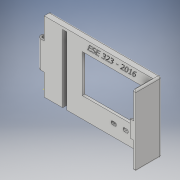
# Autodesk Inventor part: case top_new
Saved by Autodesk Inventor 2017 (Build 210142000, 142)
## iProperties
Created: 2016-12-08
Part Number: case top_new
Material: Generic
Document SubType Name: Modeling
Designer: radrajith
Density: 1 g/cm^3
Appearance: Default
Author: radrajith
Autodesk Inventor part; units mm, degrees
ref_plane "YZ Plane" through (0, 0, 0) normal (1, 0, 0) x (0, 1, 0)
ref_plane "XZ Plane" through (0, 0, 0) normal (0, 1, 0) x (-1, 0, 0)
ref_plane "XY Plane" through (0, 0, 0) normal (0, 0, 1) x (1, 0, 0)
sketch "Sketch1" plane through (0, 0, 0) normal (0, 0, 1) x (1, 0, 0)
  line L0 (0, 0) -> (138.5, 0)
  line L1 (138.5, 0) -> (138.5, 83)
  line L2 (138.5, 83) -> (0, 83)
  line L3 (0, 83) -> (0, 0)
  dimension "d0" = 138.5
  dimension "d1" = 83
  constraints: 8 end point, 2 parallel, 1 horizontal, 1 perpendicular
  measures "d0" distance of L2.end L1.end
  measures "d1" distance of L1.end L0.end
extrude "Extrusion1" add sketch "Sketch1" along normal blind 8
sketch "Sketch2" plane through (0, 0, 8) normal (0, 0, 1) x (1, 0, 0)
  line L0 (138.5, 0) -> (138.5, 83) projected
  line L1 (0, 0) -> (138.5, 0) projected
  line L2 (138.5, 83) -> (136, 83)
  line L3 (136, 83) -> (136, 0)
  line L4 (136, 0) -> (138.5, 0)
  line L5 (138.5, 0) -> (138.5, 83)
  line L6 (0, 83) -> (0, 0) projected
  dimension "d15" = 136
  constraints: 8 end point, 2 parallel, 1 horizontal, 1 perpendicular, 1 point on line
  measures "d15" distance between parallel lines of L3 L6
extrude "Extrusion2" add sketch "Sketch2" along normal blind 22.5
sketch "Sketch3" plane through (136, 0, 8) normal (-1, 0, 0) x (0, 0, 1)
  line L0 (22.5, 0) -> (22.5, 83) projected
  line L1 (22.5, 31.3) -> (20.7, 31.3)
  line L2 (20.7, 31.3) -> (20.7, 51)
  line L3 (20.7, 51) -> (22.5, 51)
  line L4 (22.5, 51) -> (22.5, 31.3)
  point P0 (-8, 0)
  dimension "d6" = 1.8
  constraints: 8 end point, 2 parallel, 1 horizontal, 1 perpendicular, 1 point on line
  measures "d6" distance of L2.end L3.end
extrude "Extrusion3" add sketch "Sketch3" along normal blind 4
sketch "Sketch5" plane through (0, 0, 8) normal (0, 0, 1) x (1, 0, 0)
  line L0 (0, 0) -> (138.5, 0) projected
  line L1 (0, 0) -> (8, 0)
  line L2 (8, 0) -> (8, 25.5)
  line L3 (8, 25.5) -> (0, 25.5)
  line L4 (0, 25.5) -> (0, 0)
  line L5 (0, 83) -> (0, 0) projected
  line L6 (0, 83) -> (8, 83)
  line L7 (8, 83) -> (8, 57.5)
  line L8 (8, 57.5) -> (0, 57.5)
  line L9 (0, 57.5) -> (0, 83)
  dimension "d9" = 8
  dimension "d10" = 25.5
  dimension "d11" = 8
  dimension "d12" = 25.5
  constraints: 16 end point, 4 parallel, 2 horizontal, 2 perpendicular
  measures "d9" distance of L3.end L2.end
  measures "d10" distance of L2.end L1.end
  measures "d11" distance of L7.end L8.end
  measures "d12" distance of L6.end L7.end
extrude "Extrusion4" cut sketch "Sketch5" against normal blind 8
sketch "Sketch6" plane through (0, 25.5, 8) normal (0, -1, 0) x (1, 0, 0)
  circle A0 centre (4, -4) radius 2
  point P0 (0, -8)
  constraints: 1 centre point
extrude "Extrusion5" cut sketch "Sketch6" against normal blind 40
fillet "Fillet1" radius 4 2 edges at (0, 41.5, 8) (0, 41.5, 0)
sketch "Sketch7" plane through (0, 0, 0) normal (0, 0, -1) x (-1, 0, 0)
  line L0 (-115, 24) -> (-53, 24)
  line L1 (-53, 24) -> (-53, 69)
  line L2 (-53, 69) -> (-115, 69)
  line L3 (-115, 69) -> (-115, 24)
  line L4 (-8, 57.5) -> (-8, 83) projected
  line L5 (-138.5, 83) -> (-8, 83) projected
  point P0 (0, 0)
  dimension "d19" = 62
  dimension "d20" = 45
  dimension "d21" = 45
  dimension "d22" = 14
  constraints: 8 end point, 2 parallel, 1 horizontal, 1 perpendicular
  measures "d19" distance of L2.end L1.end
  measures "d20" distance of L1.end L0.end
  measures "d21" distance between parallel lines of L4 L1
  measures "d22" distance between parallel lines of L2 L5
extrude "Extrusion6" cut sketch "Sketch7" against normal blind 10
chamfer "Chamfer1" distance 5 angle 45 4 edges at (115, 46.5, 0) (84, 69, 0) (53, 46.5, 0) (84, 24, 0)
sketch "Sketch8" plane through (0, 0, 8) normal (0, 0, 1) x (1, 0, 0)
  line L0 (115, 69) -> (115, 24) projected
  line L1 (115, 69) -> (125, 69)
  line L2 (125, 69) -> (125, 24)
  line L3 (125, 24) -> (115, 24)
  line L4 (115, 24) -> (115, 69)
  point P0 (0, 0)
  dimension "d28" = 10
  constraints: 8 end point, 2 parallel, 1 horizontal, 1 perpendicular
  measures "d28" distance of L2.end L3.end
extrude "Extrusion7" cut sketch "Sketch8" against normal blind 5
sketch "Sketch9" plane through (0, 0, 8) normal (0, 0, 1) x (1, 0, 0)
  line L0 (8, 0) -> (138.5, 0) projected
  line L1 (34.5, 0) -> (29.7, 0)
  line L2 (29.7, 0) -> (29.7, 80)
  line L3 (29.7, 80) -> (34.5, 80)
  line L4 (34.5, 80) -> (34.5, 0)
  point P0 (0, 0)
  dimension "d31" = 4.8
  constraints: 8 end point, 2 parallel, 1 horizontal, 1 perpendicular, 1 point on line
  measures "d31" distance of L2.end L3.end
extrude "Extrusion8" cut sketch "Sketch9" against normal blind 5
sketch "Sketch10" plane through (0, 0, 8) normal (0, 0, 1) x (1, 0, 0)
  line L0 (29.7, 0) -> (29.7, 80) projected
  line L1 (34.5, 0) -> (29.7, 0)
  line L2 (29.7, 0) -> (29.7, 10)
  line L3 (29.7, 10) -> (34.5, 10)
  line L4 (34.5, 10) -> (34.5, 0)
  point P0 (0, 0)
  constraints: 8 end point, 2 parallel, 1 horizontal, 1 perpendicular, 1 point on line
extrude "Extrusion9" cut sketch "Sketch10" against normal blind 7.2
sketch "Sketch11" plane through (0, 0, 0) normal (0, 0, -1) x (-1, 0, 0)
  line L0 (-8, 0) -> (-138.5, 0) projected
  line L1 (-136, 0) -> (-136, 83) projected
  line L2 (-105.5, 16) -> (-102.5, 16)
  line L3 (-101, 14.5) -> (-101, 13.5)
  line L4 (-102.5, 12) -> (-105.5, 12)
  line L5 (-107, 13.5) -> (-107, 14.5)
  line L6 (-107, 16) -> (-101, 12) construction
  line L7 (-101, 16) -> (-107, 12) construction
  line L8 (-91.5, 16) -> (-88.5, 16)
  line L9 (-87, 14.5) -> (-87, 13.5)
  line L10 (-88.5, 12) -> (-91.5, 12)
  line L11 (-93, 13.5) -> (-93, 14.5)
  line L12 (-93, 16) -> (-87, 12) construction
  line L13 (-87, 16) -> (-93, 12) construction
  arc A0 (-91.5, 16) -> (-93, 14.5) centre (-91.5, 14.5) ccw
  arc A1 (-93, 13.5) -> (-91.5, 12) centre (-91.5, 13.5) ccw
  arc A2 (-88.5, 12) -> (-87, 13.5) centre (-88.5, 13.5) ccw
  arc A3 (-87, 14.5) -> (-88.5, 16) centre (-88.5, 14.5) ccw
  arc A4 (-101, 14.5) -> (-102.5, 16) centre (-102.5, 14.5) ccw
  arc A5 (-105.5, 16) -> (-107, 14.5) centre (-105.5, 14.5) ccw
  arc A6 (-107, 13.5) -> (-105.5, 12) centre (-105.5, 13.5) ccw
  arc A7 (-102.5, 12) -> (-101, 13.5) centre (-102.5, 13.5) ccw
  point P0 (0, 0)
  point P1 (-104, 14)
  point P2 (-90, 14)
  dimension "d47" = 6
  dimension "d48" = 4
  dimension "d49" = 6
  dimension "d50" = 4
  dimension "d51" = 1.5
  dimension "d52" = 32
  dimension "d53" = 46
  constraints: 24 end point, 16 point on circle, 16 point on line, 16 tangent, 8 centre point, 7 equal radius, 4 midpoint, 4 parallel, 2 horizontal, 2 perpendicular
  measures "d47" distance of L6.end L7.end
  measures "d48" distance of L7.start L6.end
  measures "d49" distance of L12.end L13.end
  measures "d50" distance of L13.start L12.end
  measures "d51" radius of A0
  measures "d52" distance from line of point (-104, 14) L1
  measures "d53" distance from line of point (-90, 14) L1
extrude "Extrusion10" cut sketch "Sketch11" against normal blind 8
fillet "Fillet3" radius 2 5 edges at (138.5, 41.5, 0) (8, 70.25, 0) (73.25, 83, 0) (73.25, 0, 0) (8, 12.75, 0)
fillet "Fillet4" radius 2 6 edges at (137.25, 83, 30.5) (137.25, 0, 30.5) (137.9142, 82.4142, 0.5858) (138.5, 83, 16.25) (137.9142, 0.5858, 0.5858) (138.5, 0, 16.25)
sketch "Sketch13" plane through (0, 0, 0) normal (0, 0, -1) x (-1, 0, 0)
  point P0 (0, 0)
sketch "Sketch14" plane through (0, 0, 8) normal (0, 0, 1) x (1, 0, 0)
  line L0 (58.5434, 79.9566) -> (118.1939, 79.9566) construction
  line L1 (118.1939, 79.9566) -> (118.1939, 26.2047) construction
  line L2 (118.1939, 26.2047) -> (58.5434, 26.2047) construction
  line L3 (58.5434, 26.2047) -> (58.5434, 79.9566) construction
  line L4 (59.1613, 73.728) -> (61.2326, 79.828)
  line L5 (61.2326, 79.828) -> (65.0488, 79.828)
  line L6 (65.0488, 79.828) -> (64.8066, 79.1063)
  line L7 (64.8066, 79.1063) -> (61.8011, 79.1063)
  line L8 (61.8011, 79.1063) -> (61.2326, 77.4355)
  line L9 (61.2326, 77.4355) -> (64.0354, 77.4355)
  line L10 (64.0354, 77.4355) -> (63.7883, 76.7138)
  line L11 (63.7883, 76.7138) -> (60.9854, 76.7138)
  line L12 (60.9854, 76.7138) -> (60.2192, 74.4498)
  line L13 (60.2192, 74.4498) -> (63.2247, 74.4498)
  line L14 (63.2247, 74.4498) -> (62.9776, 73.728)
  line L15 (62.9776, 73.728) -> (59.1613, 73.728)
  spline S0 degree 2 poles (65.5332, 73.6193) (64.8659, 73.6193) (64.0305, 73.8961) (63.6894, 74.0938) knots 0 0 0 1 2 2 2
  line L16 (63.6894, 74.0938) -> (64.0354, 75.1122)
  line L17 (64.0354, 75.1122) -> (64.0947, 75.1122)
  spline S1 degree 2 poles (64.0947, 75.1122) (64.3666, 74.7365) (65.2416, 74.3212) (65.7112, 74.3212) knots 0 0 0 1 2 2 2
  spline S2 degree 2 poles (65.7112, 74.3212) (66.3835, 74.3212) (67.2584, 74.8798) (67.4166, 75.3395) knots 0 0 0 1 2 2 2
  spline S3 degree 2 poles (67.4166, 75.3395) (67.5402, 75.7053) (67.3375, 76.1601) (66.9816, 76.2738) knots 0 0 0 1 2 2 2
  spline S4 degree 2 poles (66.9816, 76.2738) (66.7246, 76.3529) (66.2945, 76.4617) (65.9732, 76.5506) knots 0 0 0 1 2 2 2
  spline S5 degree 2 poles (65.9732, 76.5506) (65.6865, 76.6347) (65.2712, 76.8868) (65.1526, 77.0895) knots 0 0 0 1 2 2 2
  spline S6 degree 2 poles (65.1526, 77.0895) (65.029, 77.2921) (65.0043, 77.8359) (65.1279, 78.1918) knots 0 0 0 1 2 2 2
  spline S7 degree 2 poles (65.1279, 78.1918) (65.38, 78.9333) (66.8729, 79.9368) (67.7725, 79.9368) knots 0 0 0 1 2 2 2
  spline S8 degree 2 poles (67.7725, 79.9368) (68.2817, 79.9368) (69.127, 79.7341) (69.4532, 79.5413) knots 0 0 0 1 2 2 2
  line L18 (69.4532, 79.5413) -> (69.122, 78.5724)
  line L19 (69.122, 78.5724) -> (69.0627, 78.5724)
  spline S9 degree 2 poles (69.0627, 78.5724) (68.8601, 78.8394) (68.0889, 79.2348) (67.5896, 79.2348) knots 0 0 0 1 2 2 2
  spline S10 degree 2 poles (67.5896, 79.2348) (67.0212, 79.2348) (66.1462, 78.7059) (66.0028, 78.2758) knots 0 0 0 1 2 2 2
  spline S11 degree 2 poles (66.0028, 78.2758) (65.8694, 77.8903) (66.1215, 77.4305) (66.4724, 77.3267) knots 0 0 0 1 2 2 2
  spline S12 degree 2 poles (66.4724, 77.3267) (66.7097, 77.2575) (67.3919, 77.0796) (67.6143, 77.0054) knots 0 0 0 1 2 2 2
  spline S13 degree 2 poles (67.6143, 77.0054) (68.1779, 76.8126) (68.4992, 76.0365) (68.3015, 75.4681) knots 0 0 0 1 2 2 2
  spline S14 degree 2 poles (68.3015, 75.4681) (68.1828, 75.1072) (67.6539, 74.4152) (67.3128, 74.1729) knots 0 0 0 1 2 2 2
  spline S15 degree 2 poles (67.3128, 74.1729) (66.9272, 73.906) (66.0869, 73.6193) (65.5332, 73.6193) knots 0 0 0 1 2 2 2
  line L20 (68.5387, 73.728) -> (70.61, 79.828)
  line L21 (70.61, 79.828) -> (74.4262, 79.828)
  line L22 (74.4262, 79.828) -> (74.184, 79.1063)
  line L23 (74.184, 79.1063) -> (71.1784, 79.1063)
  line L24 (71.1784, 79.1063) -> (70.61, 77.4355)
  line L25 (70.61, 77.4355) -> (73.4128, 77.4355)
  line L26 (73.4128, 77.4355) -> (73.1656, 76.7138)
  line L27 (73.1656, 76.7138) -> (70.3628, 76.7138)
  line L28 (70.3628, 76.7138) -> (69.5966, 74.4498)
  line L29 (69.5966, 74.4498) -> (72.6021, 74.4498)
  line L30 (72.6021, 74.4498) -> (72.3549, 73.728)
  line L31 (72.3549, 73.728) -> (68.5387, 73.728)
  spline S16 degree 2 poles (79.2113, 79.2497) (78.9938, 79.2497) (78.5143, 79.1409) (78.272, 79.0569) knots 0 0 0 1 2 2 2
  spline S17 degree 2 poles (78.272, 79.0569) (78.0496, 78.9729) (77.6937, 78.7949) (77.5553, 78.7158) knots 0 0 0 1 2 2 2
  line L32 (77.5553, 78.7158) -> (77.5058, 78.7158)
  line L33 (77.5058, 78.7158) -> (77.7975, 79.5809)
  spline S18 degree 2 poles (77.7975, 79.5809) (78.1139, 79.7242) (79.1075, 79.9566) (79.5227, 79.9566) knots 0 0 0 1 2 2 2
  spline S19 degree 2 poles (79.5227, 79.9566) (79.933, 79.9566) (80.4965, 79.7885) (80.6844, 79.6105) knots 0 0 0 1 2 2 2
  spline S20 degree 2 poles (80.6844, 79.6105) (80.887, 79.4177) (80.976, 78.8592) (80.8475, 78.4835) knots 0 0 0 1 2 2 2
  spline S21 degree 2 poles (80.8475, 78.4835) (80.6745, 77.9793) (79.755, 77.218) (79.2558, 77.1191) knots 0 0 0 1 2 2 2
  line L34 (79.2558, 77.1191) -> (79.236, 77.0598)
  spline S22 degree 2 poles (79.236, 77.0598) (79.4189, 77.0203) (79.7946, 76.8423) (79.9231, 76.6643) knots 0 0 0 1 2 2 2
  spline S23 degree 2 poles (79.9231, 76.6643) (80.0516, 76.4913) (80.1011, 75.9377) (79.9626, 75.5373) knots 0 0 0 1 2 2 2
  spline S24 degree 2 poles (79.9626, 75.5373) (79.8242, 75.127) (79.3052, 74.43) (78.9592, 74.163) knots 0 0 0 1 2 2 2
  spline S25 degree 2 poles (78.9592, 74.163) (78.5983, 73.8862) (77.7431, 73.5995) (77.2636, 73.5995) knots 0 0 0 1 2 2 2
  spline S26 degree 2 poles (77.2636, 73.5995) (76.8088, 73.5995) (75.9833, 73.822) (75.7263, 73.9752) knots 0 0 0 1 2 2 2
  line L35 (75.7263, 73.9752) -> (76.0179, 74.8403)
  line L36 (76.0179, 74.8403) -> (76.0772, 74.8403)
  spline S27 degree 2 poles (76.0772, 74.8403) (76.27, 74.6524) (77.0214, 74.3064) (77.4564, 74.3064) knots 0 0 0 1 2 2 2
  spline S28 degree 2 poles (77.4564, 74.3064) (77.7085, 74.3064) (78.2671, 74.4646) (78.4945, 74.6475) knots 0 0 0 1 2 2 2
  spline S29 degree 2 poles (78.4945, 74.6475) (78.7219, 74.8304) (79.0432, 75.2654) (79.1569, 75.5966) knots 0 0 0 1 2 2 2
  spline S30 degree 2 poles (79.1569, 75.5966) (79.2656, 75.9278) (79.2212, 76.3579) (79.0877, 76.4814) knots 0 0 0 1 2 2 2
  spline S31 degree 2 poles (79.0877, 76.4814) (78.9592, 76.605) (78.5192, 76.6989) (78.2473, 76.6989) knots 0 0 0 1 2 2 2
  line L37 (78.2473, 76.6989) -> (77.8964, 76.6989)
  line L38 (77.8964, 76.6989) -> (78.1287, 77.3762)
  line L39 (78.1287, 77.3762) -> (78.3956, 77.3762)
  spline S32 degree 2 poles (78.3956, 77.3762) (78.9493, 77.3762) (79.8193, 77.9002) (79.9874, 78.3994) knots 0 0 0 1 2 2 2
  spline S33 degree 2 poles (79.9874, 78.3994) (80.0665, 78.6318) (79.9972, 78.963) (79.8934, 79.0618) knots 0 0 0 1 2 2 2
  spline S34 degree 2 poles (79.8934, 79.0618) (79.7748, 79.1656) (79.4238, 79.2497) (79.2113, 79.2497) knots 0 0 0 1 2 2 2
  line L40 (84.031, 73.728) -> (80.2691, 73.728)
  line L41 (80.2691, 73.728) -> (80.5608, 74.5931)
  spline S35 degree 2 poles (80.5608, 74.5931) (81.0996, 74.9737) (82.0586, 75.6806) (82.5331, 76.0613) knots 0 0 0 1 2 2 2
  spline S36 degree 2 poles (82.5331, 76.0613) (83.4921, 76.8275) (84.3127, 77.7469) (84.4808, 78.2363) knots 0 0 0 1 2 2 2
  spline S37 degree 2 poles (84.4808, 78.2363) (84.5698, 78.4934) (84.5401, 78.8789) (84.4413, 79.0025) knots 0 0 0 1 2 2 2
  spline S38 degree 2 poles (84.4413, 79.0025) (84.3424, 79.1261) (84.0062, 79.2497) (83.7789, 79.2497) knots 0 0 0 1 2 2 2
  spline S39 degree 2 poles (83.7789, 79.2497) (83.5613, 79.2497) (83.0769, 79.1409) (82.8446, 79.0569) knots 0 0 0 1 2 2 2
  spline S40 degree 2 poles (82.8446, 79.0569) (82.6468, 78.9877) (82.2613, 78.7899) (82.1377, 78.7207) knots 0 0 0 1 2 2 2
  line L42 (82.1377, 78.7207) -> (82.0932, 78.7207)
  line L43 (82.0932, 78.7207) -> (82.3898, 79.5908)
  spline S41 degree 2 poles (82.3898, 79.5908) (82.6864, 79.7143) (83.675, 79.9566) (84.0804, 79.9566) knots 0 0 0 1 2 2 2
  spline S42 degree 2 poles (84.0804, 79.9566) (84.9306, 79.9566) (85.5881, 79.0519) (85.3261, 78.2808) knots 0 0 0 1 2 2 2
  spline S43 degree 2 poles (85.3261, 78.2808) (85.2025, 77.9199) (84.8318, 77.3169) (84.5945, 77.0598) knots 0 0 0 1 2 2 2
  spline S44 degree 2 poles (84.5945, 77.0598) (84.3523, 76.7929) (83.7492, 76.2689) (83.4279, 76.0168) knots 0 0 0 1 2 2 2
  spline S45 degree 2 poles (83.4279, 76.0168) (82.8989, 75.5966) (81.6483, 74.6969) (81.2776, 74.4349) knots 0 0 0 1 2 2 2
  line L44 (81.2776, 74.4349) -> (84.2732, 74.4349)
  line L45 (84.2732, 74.4349) -> (84.031, 73.728)
  spline S46 degree 2 poles (88.3662, 79.2497) (88.1487, 79.2497) (87.6692, 79.1409) (87.427, 79.0569) knots 0 0 0 1 2 2 2
  spline S47 degree 2 poles (87.427, 79.0569) (87.2045, 78.9729) (86.8486, 78.7949) (86.7102, 78.7158) knots 0 0 0 1 2 2 2
  line L46 (86.7102, 78.7158) -> (86.6608, 78.7158)
  line L47 (86.6608, 78.7158) -> (86.9524, 79.5809)
  spline S48 degree 2 poles (86.9524, 79.5809) (87.2688, 79.7242) (88.2624, 79.9566) (88.6776, 79.9566) knots 0 0 0 1 2 2 2
  spline S49 degree 2 poles (88.6776, 79.9566) (89.0879, 79.9566) (89.6515, 79.7885) (89.8393, 79.6105) knots 0 0 0 1 2 2 2
  spline S50 degree 2 poles (89.8393, 79.6105) (90.042, 79.4177) (90.131, 78.8592) (90.0024, 78.4835) knots 0 0 0 1 2 2 2
  spline S51 degree 2 poles (90.0024, 78.4835) (89.8294, 77.9793) (88.91, 77.218) (88.4107, 77.1191) knots 0 0 0 1 2 2 2
  line L48 (88.4107, 77.1191) -> (88.3909, 77.0598)
  spline S52 degree 2 poles (88.3909, 77.0598) (88.5738, 77.0203) (88.9495, 76.8423) (89.078, 76.6643) knots 0 0 0 1 2 2 2
  spline S53 degree 2 poles (89.078, 76.6643) (89.2066, 76.4913) (89.256, 75.9377) (89.1176, 75.5373) knots 0 0 0 1 2 2 2
  spline S54 degree 2 poles (89.1176, 75.5373) (88.9792, 75.127) (88.4601, 74.43) (88.1141, 74.163) knots 0 0 0 1 2 2 2
  spline S55 degree 2 poles (88.1141, 74.163) (87.7532, 73.8862) (86.8981, 73.5995) (86.4186, 73.5995) knots 0 0 0 1 2 2 2
  spline S56 degree 2 poles (86.4186, 73.5995) (85.9638, 73.5995) (85.1383, 73.822) (84.8812, 73.9752) knots 0 0 0 1 2 2 2
  line L49 (84.8812, 73.9752) -> (85.1729, 74.8403)
  line L50 (85.1729, 74.8403) -> (85.2322, 74.8403)
  spline S57 degree 2 poles (85.2322, 74.8403) (85.425, 74.6524) (86.1763, 74.3064) (86.6113, 74.3064) knots 0 0 0 1 2 2 2
  spline S58 degree 2 poles (86.6113, 74.3064) (86.8635, 74.3064) (87.422, 74.4646) (87.6494, 74.6475) knots 0 0 0 1 2 2 2
  spline S59 degree 2 poles (87.6494, 74.6475) (87.8768, 74.8304) (88.1981, 75.2654) (88.3118, 75.5966) knots 0 0 0 1 2 2 2
  spline S60 degree 2 poles (88.3118, 75.5966) (88.4206, 75.9278) (88.3761, 76.3579) (88.2426, 76.4814) knots 0 0 0 1 2 2 2
  spline S61 degree 2 poles (88.2426, 76.4814) (88.1141, 76.605) (87.6742, 76.6989) (87.4023, 76.6989) knots 0 0 0 1 2 2 2
  line L51 (87.4023, 76.6989) -> (87.0513, 76.6989)
  line L52 (87.0513, 76.6989) -> (87.2836, 77.3762)
  line L53 (87.2836, 77.3762) -> (87.5506, 77.3762)
  spline S62 degree 2 poles (87.5506, 77.3762) (88.1042, 77.3762) (88.9742, 77.9002) (89.1423, 78.3994) knots 0 0 0 1 2 2 2
  spline S63 degree 2 poles (89.1423, 78.3994) (89.2214, 78.6318) (89.1522, 78.963) (89.0484, 79.0618) knots 0 0 0 1 2 2 2
  spline S64 degree 2 poles (89.0484, 79.0618) (88.9297, 79.1656) (88.5788, 79.2497) (88.3662, 79.2497) knots 0 0 0 1 2 2 2
  line L54 (95.0594, 76.0267) -> (92.7509, 76.0267)
  line L55 (92.7509, 76.0267) -> (93.003, 76.7682)
  line L56 (93.003, 76.7682) -> (95.3115, 76.7682)
  line L57 (95.3115, 76.7682) -> (95.0594, 76.0267)
  line L58 (101.4708, 73.728) -> (97.709, 73.728)
  line L59 (97.709, 73.728) -> (98.0007, 74.5931)
  spline S65 degree 2 poles (98.0007, 74.5931) (98.5395, 74.9737) (99.4985, 75.6806) (99.973, 76.0613) knots 0 0 0 1 2 2 2
  spline S66 degree 2 poles (99.973, 76.0613) (100.932, 76.8275) (101.7526, 77.7469) (101.9207, 78.2363) knots 0 0 0 1 2 2 2
  spline S67 degree 2 poles (101.9207, 78.2363) (102.0096, 78.4934) (101.98, 78.8789) (101.8811, 79.0025) knots 0 0 0 1 2 2 2
  spline S68 degree 2 poles (101.8811, 79.0025) (101.7823, 79.1261) (101.4461, 79.2497) (101.2187, 79.2497) knots 0 0 0 1 2 2 2
  spline S69 degree 2 poles (101.2187, 79.2497) (101.0012, 79.2497) (100.5168, 79.1409) (100.2844, 79.0569) knots 0 0 0 1 2 2 2
  spline S70 degree 2 poles (100.2844, 79.0569) (100.0867, 78.9877) (99.7011, 78.7899) (99.5776, 78.7207) knots 0 0 0 1 2 2 2
  line L60 (99.5776, 78.7207) -> (99.5331, 78.7207)
  line L61 (99.5331, 78.7207) -> (99.8297, 79.5908)
  spline S71 degree 2 poles (99.8297, 79.5908) (100.1263, 79.7143) (101.1149, 79.9566) (101.5203, 79.9566) knots 0 0 0 1 2 2 2
  spline S72 degree 2 poles (101.5203, 79.9566) (102.3705, 79.9566) (103.028, 79.0519) (102.766, 78.2808) knots 0 0 0 1 2 2 2
  spline S73 degree 2 poles (102.766, 78.2808) (102.6424, 77.9199) (102.2716, 77.3169) (102.0344, 77.0598) knots 0 0 0 1 2 2 2
  spline S74 degree 2 poles (102.0344, 77.0598) (101.7921, 76.7929) (101.1891, 76.2689) (100.8677, 76.0168) knots 0 0 0 1 2 2 2
  spline S75 degree 2 poles (100.8677, 76.0168) (100.3388, 75.5966) (99.0882, 74.6969) (98.7174, 74.4349) knots 0 0 0 1 2 2 2
  line L62 (98.7174, 74.4349) -> (101.713, 74.4349)
  line L63 (101.713, 74.4349) -> (101.4708, 73.728)
  spline S76 degree 2 poles (107.121, 76.778) (106.5624, 75.1369) (105.0844, 73.5995) (104.0908, 73.5995) knots 0 0 0 1 2 2 2
  spline S77 degree 2 poles (104.0908, 73.5995) (103.0823, 73.5995) (102.672, 75.1665) (103.2158, 76.7731) knots 0 0 0 1 2 2 2
  spline S78 degree 2 poles (103.2158, 76.7731) (103.7793, 78.4241) (105.2524, 79.9516) (106.246, 79.9516) knots 0 0 0 1 2 2 2
  spline S79 degree 2 poles (106.246, 79.9516) (107.2545, 79.9516) (107.6598, 78.3698) (107.121, 76.778) knots 0 0 0 1 2 2 2
  spline S80 degree 2 poles (105.4403, 74.9194) (105.6627, 75.2209) (106.073, 76.1502) (106.2905, 76.778) knots 0 0 0 1 2 2 2
  spline S81 degree 2 poles (106.2905, 76.778) (106.5031, 77.4058) (106.7206, 78.3302) (106.7008, 78.6417) knots 0 0 0 1 2 2 2
  spline S82 degree 2 poles (106.7008, 78.6417) (106.681, 78.9531) (106.3647, 79.2744) (106.0186, 79.2744) knots 0 0 0 1 2 2 2
  spline S83 degree 2 poles (106.0186, 79.2744) (105.6776, 79.2744) (105.1289, 78.9531) (104.8916, 78.6318) knots 0 0 0 1 2 2 2
  spline S84 degree 2 poles (104.8916, 78.6318) (104.6642, 78.3203) (104.2489, 77.3712) (104.0463, 76.7731) knots 0 0 0 1 2 2 2
  spline S85 degree 2 poles (104.0463, 76.7731) (103.8288, 76.1305) (103.6162, 75.2703) (103.631, 74.9342) knots 0 0 0 1 2 2 2
  spline S86 degree 2 poles (103.631, 74.9342) (103.6409, 74.6178) (103.9672, 74.2767) (104.3182, 74.2767) knots 0 0 0 1 2 2 2
  spline S87 degree 2 poles (104.3182, 74.2767) (104.6592, 74.2767) (105.2079, 74.5981) (105.4403, 74.9194) knots 0 0 0 1 2 2 2
  line L64 (110.3193, 73.728) -> (107.3434, 73.728)
  line L65 (107.3434, 73.728) -> (107.556, 74.3509)
  line L66 (107.556, 74.3509) -> (108.6633, 74.3509)
  line L67 (108.6633, 74.3509) -> (110.0524, 78.439)
  line L68 (110.0524, 78.439) -> (108.9451, 78.439)
  line L69 (108.9451, 78.439) -> (109.1329, 78.9976)
  spline S88 degree 2 poles (109.1329, 78.9976) (109.7607, 78.9976) (110.4775, 79.3535) (110.6801, 79.8478) knots 0 0 0 1 2 2 2
  line L70 (110.6801, 79.8478) -> (111.3178, 79.8478)
  line L71 (111.3178, 79.8478) -> (109.4493, 74.3509)
  line L72 (109.4493, 74.3509) -> (110.5319, 74.3509)
  line L73 (110.5319, 74.3509) -> (110.3193, 73.728)
  spline S89 degree 2 poles (115.9695, 75.7053) (115.8113, 75.2357) (115.228, 74.4399) (114.877, 74.1729) knots 0 0 0 1 2 2 2
  spline S90 degree 2 poles (114.877, 74.1729) (114.5062, 73.8912) (113.7252, 73.5995) (113.3149, 73.5995) knots 0 0 0 1 2 2 2
  spline S91 degree 2 poles (113.3149, 73.5995) (112.9046, 73.5995) (112.3213, 73.8763) (112.1582, 74.1532) knots 0 0 0 1 2 2 2
  spline S92 degree 2 poles (112.1582, 74.1532) (111.9555, 74.4844) (111.9753, 75.5966) (112.2521, 76.4073) knots 0 0 0 1 2 2 2
  spline S93 degree 2 poles (112.2521, 76.4073) (112.524, 77.2032) (113.2853, 78.4835) (113.7895, 78.958) knots 0 0 0 1 2 2 2
  spline S94 degree 2 poles (113.7895, 78.958) (114.2739, 79.4227) (115.4998, 79.9417) (116.187, 79.9417) knots 0 0 0 1 2 2 2
  spline S95 degree 2 poles (116.187, 79.9417) (116.3946, 79.9417) (116.7307, 79.9022) (116.8494, 79.8577) knots 0 0 0 1 2 2 2
  line L74 (116.8494, 79.8577) -> (116.5824, 79.0717)
  line L75 (116.5824, 79.0717) -> (116.5478, 79.0717)
  spline S96 degree 2 poles (116.5478, 79.0717) (116.4588, 79.131) (116.0733, 79.2348) (115.8409, 79.2348) knots 0 0 0 1 2 2 2
  spline S97 degree 2 poles (115.8409, 79.2348) (115.0797, 79.2348) (113.7944, 78.2066) (113.3643, 77.1982) knots 0 0 0 1 2 2 2
  spline S98 degree 2 poles (113.3643, 77.1982) (113.7252, 77.4009) (114.4123, 77.6233) (114.7781, 77.6233) knots 0 0 0 1 2 2 2
  spline S99 degree 2 poles (114.7781, 77.6233) (115.134, 77.6233) (115.6185, 77.48) (115.836, 77.2625) knots 0 0 0 1 2 2 2
  spline S100 degree 2 poles (115.836, 77.2625) (116.0831, 77.0104) (116.1474, 76.2293) (115.9695, 75.7053) knots 0 0 0 1 2 2 2
  spline S101 degree 2 poles (115.1291, 75.6707) (115.2527, 76.0464) (115.2329, 76.5556) (115.0698, 76.7335) knots 0 0 0 1 2 2 2
  spline S102 degree 2 poles (115.0698, 76.7335) (114.9561, 76.8621) (114.5804, 76.9461) (114.3678, 76.9461) knots 0 0 0 1 2 2 2
  spline S103 degree 2 poles (114.3678, 76.9461) (114.0811, 76.9461) (113.483, 76.7731) (113.1617, 76.61) knots 0 0 0 1 2 2 2
  spline S104 degree 2 poles (113.1617, 76.61) (113.1271, 76.521) (113.0579, 76.3529) (113.0183, 76.2244) knots 0 0 0 1 2 2 2
  spline S105 degree 2 poles (113.0183, 76.2244) (112.8008, 75.5917) (112.786, 74.8156) (112.9046, 74.6129) knots 0 0 0 1 2 2 2
  spline S106 degree 2 poles (112.9046, 74.6129) (113.0134, 74.4201) (113.3347, 74.2669) (113.5472, 74.2669) knots 0 0 0 1 2 2 2
  spline S107 degree 2 poles (113.5472, 74.2669) (114.0416, 74.2669) (114.8869, 74.9688) (115.1291, 75.6707) knots 0 0 0 1 2 2 2
  point P0 (0, 0)
  constraints: 2 other
extrude "Extrusion12" cut sketch "Sketch14" against normal blind 2
body "Solid1"
